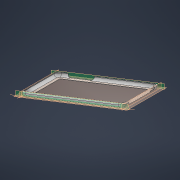
# Autodesk Inventor part: test_fit1
Saved by Autodesk Inventor 2021 (Build 250183000, 183)
## iProperties
Created: 2020-09-27
Part Number: test_fit1
Material: Generic
Document SubType Name: Modeling
Designer: brand
Density: 1 g/cm^3
Appearance: Default
Author: brand
Autodesk Inventor part; units mm, degrees
sketch "Sketch1" plane through (0, 0, 0) normal (0, 0, 1) x (1, 0, 0)
  line L0 (0, 0) -> (208.4, 0)
  line L1 (208.4, 0) -> (208.4, 137.5)
  line L2 (208.4, 137.5) -> (0, 137.5)
  line L3 (0, 137.5) -> (0, 0)
  dimension "d0" = 208.4
  dimension "d1" = 137.5
  constraints: 8 end point, 2 parallel, 1 horizontal, 1 perpendicular
  measures "d0" distance of L1.end L2.end
  measures "d1" distance of L0.end L1.end
extrude "Extrusion1" add sketch "Sketch1" along normal blind 7.9
fillet "Fillet1" radius 9.9 4 edges at (0, 137.5, 3.95) (0, 0, 3.95) (208.4, 0, 3.95) (208.4, 137.5, 3.95)
fillet "Fillet2" radius 2 8 edges at (205.5004, 2.8996, 7.9) (208.4, 68.75, 7.9) (205.5004, 134.6004, 7.9) (104.2, 137.5, 7.9) (2.8996, 134.6004, 7.9) (0, 68.75, 7.9) (2.8996, 2.8996, 7.9) (104.2, 0, 7.9)
fillet "Fillet3" radius 5.9 8 edges at (205.5004, 2.8996, 0) (208.4, 68.75, 0) (205.5004, 134.6004, 0) (104.2, 137.5, 0) (2.8996, 134.6004, 0) (0, 68.75, 0) (2.8996, 2.8996, 0) (104.2, 0, 0)
thicken "Thicken1" operation new thickness 0.8 both sides no extend neighbours no toward (-0.9972038, -0.0747301, 0) faces at (0.027682, 9.160172, 5.899933) (0.116105, 8.425315, 6.04946) (72.766667, 0, 5.899933) (72.766667, 0.639655, 7.366104) (202.116876, 0.68435, 5.899933) (208.283895, 8.425315, 6.04946) (208.4, 88.366667, 5.899967) (206.54946, 49.133333, 7.894408) (199.974685, 137.383895, 6.04946) (208.372318, 128.339828, 5.899933) (135.633333, 135.64946, 7.894408) (72.766667, 137.5, 5.899967) (9.160172, 137.472318, 5.899933) (8.425315, 137.383895, 6.04946) (0, 49.133333, 5.899933) (0.533896, 88.366667, 7.260345) (0.065897, 88.366667, 5.020566) (1.1046, 5.501076, 5.020566) (72.766667, 0.016497, 5.459) (202.898924, 1.1046, 5.020566) (204.655576, 49.133333, 0.407838) (207.2954, 131.998924, 5.020566) (72.766667, 133.339126, 0.262116) (1.1046, 131.998924, 5.020566) (72.766667, 89.700033, 0)
sketch "Sketch3" plane through (9.9, 131.6, 0) normal (0, 0, 1) x (1, 0, 0)
  line L0 (4, -113.7) -> (4, -12)
  arc A0 (8, -8) -> (4, -12) centre (8, -12) ccw
  line L1 (8, -8) -> (180.6, -8)
  arc A1 (184.6, -12) -> (180.6, -8) centre (180.6, -12) ccw
  line L2 (184.6, -12) -> (184.6, -113.7)
  line L3 (180.6, -117.7) -> (8, -117.7)
  arc A2 (4, -113.7) -> (8, -117.7) centre (8, -113.7) ccw
  arc A3 (-4, -121.7) -> (0, -125.7) centre (0, -121.7) ccw projected
  arc A4 (180.6, -117.7) -> (184.6, -113.7) centre (180.6, -113.7) ccw
  line L4 (-4, -4) -> (-4, -121.7) projected
  line L5 (188.6, 0) -> (0, 0) projected
  line L6 (192.6, -121.7) -> (192.6, -4) projected
  line L7 (188.6, -129.6) -> (0, -129.6) projected
  line L8 (0, -125.7) -> (188.6, -125.7) projected
  point P0 (-9.9, -131.6)
  dimension "middle_cutout" = 8
  dimension "d14" = 8
  dimension "d15" = 8
  dimension "d17" = 8
  constraints: 8 end point, 8 point on circle, 7 tangent, 4 centre point, 3 equal radius, 2 horizontal, 2 parallel, 2 vertical
  measures "middle_cutout" distance between parallel lines of L4 L0
  measures "d14" distance between parallel lines of L5 L1
  measures "d15" distance between parallel lines of L6 L2
  measures "d17" distance between parallel lines of L8 L3
extrude "Extrusion2" cut sketch "Sketch3" against normal through all bodies 2
ref_plane "Work Plane1" through (198.5, 138.3, 5.9) normal (0, 1, 0) x (-1, 0, 0)
sketch "Sketch4" plane through (198.5, 138.3, 5.9) normal (0, 1, 0) x (-1, 0, 0)
  line L0 (188.6, 2.8) -> (0, 2.8) projected
  line L1 (0, -5.9) -> (188.6, -5.9) projected
  line L2 (174.8, 2.8) -> (121.3, 2.8)
  line L3 (121.3, 2.8) -> (121.3, -5.9)
  line L4 (121.3, -5.9) -> (174.8, -5.9)
  line L5 (174.8, -5.9) -> (174.8, 2.8)
  arc A0 (168.9, -5.9) -> (174.8, 0) centre (168.9, 0) ccw
  arc A1 (121.3, 0) -> (127.2, -5.9) centre (127.2, 0) ccw
  point P0 (198.5, -5.9)
  point P1 (199.3, 0)
  point P2 (127.2, -5.9)
  point P3 (168.9, -5.9)
  dimension "d20" = 53.5
  dimension "d21" = 24.5
  dimension "d31" = 5.9
  constraints: 8 end point, 6 point on line, 4 point on circle, 4 tangent, 2 centre point, 2 parallel, 1 equal radius, 1 horizontal, 1 perpendicular
  measures "d20" distance between parallel lines of L5 L3
  measures "d21" distance from line of point (199.3, 0) L5
  measures "d31" radius of A0
extrude "Extrusion3" cut sketch "Sketch4" against normal blind 10 contours L5 A0 L1 A1 L3 L0 bodies 2
ref_plane "Work Plane2" through (209.2, 127.6, 5.9) normal (1, 0, 0) x (0, 1, 0)
sketch "Sketch5" plane through (209.2, 127.6, 5.9) normal (1, 0, 0) x (0, 1, 0)
  line L0 (0, 2.8) -> (-117.7, 2.8) projected
  line L1 (-109.7, -5.9) -> (-8, -5.9) projected
  line L2 (-109.4, 2.8) -> (-8.3, 2.8)
  line L3 (-8.3, 2.8) -> (-8.3, -5.9)
  line L4 (-8.3, -5.9) -> (-109.4, -5.9)
  line L5 (-109.4, -5.9) -> (-109.4, 2.8)
  line L6 (0, -5.9) -> (-117.7, -5.9) projected
  arc A0 (-109.4, 0) -> (-103.5, -5.9) centre (-103.5, 0) ccw
  arc A1 (-14.2, -5.9) -> (-8.3, 0) centre (-14.2, 0) ccw
  point P0 (-127.6, -5.9)
  point P1 (-128.4, 0)
  point P2 (10.7, 0)
  point P3 (-103.5, -5.9)
  dimension "d24" = 19
  dimension "d25" = 19
  dimension "d28" = 5.9
  constraints: 8 end point, 6 point on line, 4 point on circle, 4 tangent, 2 centre point, 2 parallel, 1 equal radius, 1 horizontal, 1 perpendicular
  measures "d24" distance from line of point (-128.4, 0) L5
  measures "d25" distance from line of point (10.7, 0) L3
  measures "d28" radius of A0
extrude "Extrusion5" cut sketch "Sketch5" against normal blind 10 contours L3 A1 L1 A0 L5 L0 bodies 2
equation "\"d6\" = D - chrome_edge"
equation "\"d14\" = middle_cutout"
equation "\"d15\" = middle_cutout"
equation "\"d17\" = middle_cutout"
equation "\"d31\" = D - chrome_edge"
equation "\"d25\" = d24"
equation "\"d28\" = D - chrome_edge"
equation "\"D\" = 7.9"
equation "\"chrome_edge\" = 2"
body "Solid1"
body "Solid2"
